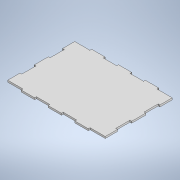
# Autodesk Inventor part: base
Saved by Autodesk Inventor 2020 (Build 240168000, 168)
## iProperties
Created: 2020-02-22
Part Number: base
Material: Generic
Document SubType Name: Modeling
Designer: udvarhelyi
Density: 1 g/cm^3
Appearance: Default
Author: udvarhelyi
Autodesk Inventor part; units mm, degrees
ref_plane "YZ Plane" through (0, 0, 0) normal (1, 0, 0) x (0, 1, 0)
ref_plane "XZ Plane" through (0, 0, 0) normal (0, 1, 0) x (-1, 0, 0)
ref_plane "XY Plane" through (0, 0, 0) normal (0, 0, 1) x (1, 0, 0)
sketch "Sketch1" plane through (0, 0, 0) normal (0, 1, 0) x (-1, 0, 0)
  line L0 (-11.4286, -54) -> (-11.4286, -57)
  line L1 (-11.4286, -57) -> (11.4286, -57)
  line L2 (11.4286, -57) -> (11.4286, -54)
  line L3 (-57.1429, -54) -> (-57.1429, -57)
  line L4 (-57.1429, -57) -> (-34.2857, -57)
  line L5 (-34.2857, -57) -> (-34.2857, -54)
  line L6 (57.1429, -54) -> (57.1429, -57)
  line L7 (57.1429, -57) -> (34.2857, -57)
  line L8 (34.2857, -57) -> (34.2857, -54)
  line L9 (34.2857, 60) -> (34.2857, 63)
  line L10 (34.2857, 63) -> (57.1429, 63)
  line L11 (57.1429, 63) -> (57.1429, 60)
  line L12 (-11.4286, 60) -> (-11.4286, 63)
  line L13 (-11.4286, 63) -> (11.4286, 63)
  line L14 (11.4286, 63) -> (11.4286, 60)
  line L15 (-57.1429, 60) -> (-57.1429, 63)
  line L16 (-57.1429, 63) -> (-34.2857, 63)
  line L17 (-34.2857, 63) -> (-34.2857, 60)
  line L18 (80, 60) -> (83, 60)
  line L19 (83, -54) -> (80, -54)
  line L20 (-80, 60) -> (-83, 60)
  line L21 (-83, -54) -> (-80, -54)
  line L22 (80, -54) -> (80, -54)
  line L23 (80, 60) -> (80, 60)
  line L24 (57.1429, -54) -> (80, -54)
  line L25 (11.4286, -54) -> (34.2857, -54)
  line L26 (-80, -54) -> (-57.1429, -54)
  line L27 (-34.2857, -54) -> (-11.4286, -54)
  line L28 (-80, 60) -> (-80, 60)
  line L29 (-80, -54) -> (-80, -54)
  line L30 (-57.1429, 60) -> (-80, 60)
  line L31 (-11.4286, 60) -> (-34.2857, 60)
  line L32 (80, 60) -> (57.1429, 60)
  line L33 (34.2857, 60) -> (11.4286, 60)
  line L34 (83, -33) -> (80, -33)
  line L35 (80, -33) -> (80, -9)
  line L36 (80, -9) -> (83, -9)
  line L37 (83, 39) -> (80, 39)
  line L38 (80, 39) -> (80, 15)
  line L39 (80, 15) -> (83, 15)
  line L40 (-83, 39) -> (-80, 39)
  line L41 (-80, 39) -> (-80, 15)
  line L42 (-80, 15) -> (-83, 15)
  line L43 (-83, -9) -> (-80, -9)
  line L44 (-80, -9) -> (-80, -33)
  line L45 (-80, -33) -> (-83, -33)
  line L46 (83, -33) -> (83, -54)
  line L47 (83, 60) -> (83, 39)
  line L48 (83, 15) -> (83, -9)
  line L49 (-83, 60) -> (-83, 39)
  line L50 (-83, 15) -> (-83, -9)
  line L51 (-83, -33) -> (-83, -54)
  point P0 (0, 0)
  dimension "d40" = 160
  dimension "d47" = 22.8571
  dimension "d48" = 22.8571
  dimension "d49" = 3
  dimension "d50" = 3
  dimension "d51" = 3
  dimension "d52" = 3
  dimension "d53" = 3
  dimension "d54" = 3
  dimension "d55" = 80
  dimension "d56" = 60
  dimension "d57" = 114
  dimension "d58" = 0
  dimension "d59" = 0
  dimension "d61" = 24
  dimension "d62" = 24
  dimension "d63" = 24
  dimension "d64" = 3
  constraints: 104 end point, 34 parallel, 19 perpendicular, 18 collinear, 18 point on line, 10 horizontal, 7 equal length, 1 other
  measures "d40" distance of L26.start L22.start
  measures "d47" distance of L9.end L10.end
  measures "d48" distance of L9.start L14.end
  measures "d49" distance of L19.start L19.end
  measures "d50" distance of L21.start L21.end
  measures "d51" distance of L3.start L3.end
  measures "d52" distance of L15.start L15.end
  measures "d53" distance of L10.end L11.end
  measures "d54" distance of L6.start L6.end
  measures "d55" distance from line of L28 point (0, 0)
  measures "d56" distance from line of point (0, 0) L31
  measures "d57" distance between parallel lines of L30 L26
  measures "d58" distance from line of L32 L18.end
  measures "d59" distance from line of L24 L19.start
  measures "d61" distance from line of L37.start L10
  measures "d62" distance of L37.end L38.end
  measures "d63" distance of L39.end L36.end
  measures "d64" distance of L37.start L37.end
extrude "Extrusion1" add sketch "Sketch1" along normal blind 3
equation "\"d40\" = shelfW"
equation "\"d47\" = 0.142857 * shelfW + 2 * tol"
equation "\"d48\" = 0.142857 * shelfW - 2 * tol"
equation "\"d49\" = tt"
equation "\"d50\" = tt"
equation "\"d51\" = tt"
equation "\"d52\" = tt"
equation "\"d53\" = tt"
equation "\"d54\" = tt"
equation "\"d55\" = 0.5 * shelfW"
equation "\"d56\" = 0.5 * ht"
equation "\"d57\" = -2 * tt + ht"
equation "\"d61\" = 0.2 * ht - tol"
equation "\"d62\" = 0.2 * ht + 2 * tol"
equation "\"d63\" = 0.2 * ht - 2 * tol"
equation "\"d64\" = tt"
equation "\"d31\" = tt"
equation "\"d4\" = tt"
equation "\"tt\" = 3"
equation "\"tol\" = 0"
equation "\"tiroir\" = 1"
equation "\"nHoles\" = 4"
equation "\"shelfW\" = 160"
equation "\"shelfH\" = 35"
equation "\"d43\" = 0.5 * shelfH"
equation "\"ht\" = 120"
body "Solid1"
